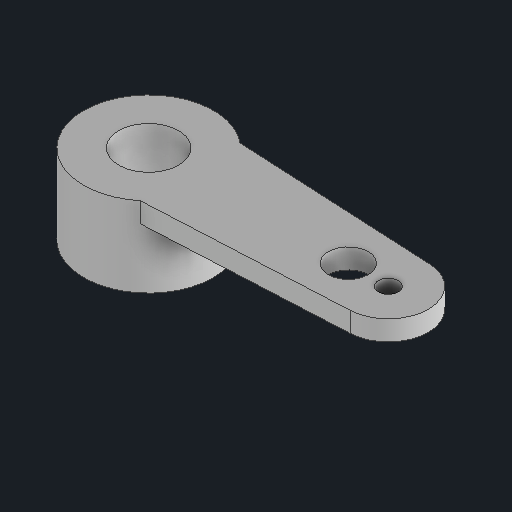
# Autodesk Inventor part: P_Servo_SIMPROP_lever
Saved by Autodesk Inventor 2026 (Build 300175000, 175)
## iProperties
Created: 2025-09-02
Part Number: P_Servo_SIMPROP_lever
Material: Generisch
Document SubType Name: Modeling
Designer: FAL
Density: 1 g/cm^3
Appearance: Vorgabe
Author: FAL
Autodesk Inventor part; units mm, degrees
ref_plane "YZ Plane" through (0, 0, 0) normal (1, 0, 0) x (0, 1, 0)
ref_plane "XZ Plane" through (0, 0, 0) normal (0, 1, 0) x (-1, 0, 0)
ref_plane "XY Plane" through (0, 0, 0) normal (0, 0, 1) x (1, 0, 0)
sketch "Skizze1" plane through (0, 0, 0) normal (0, 0, 1) x (1, 0, 0)
  circle A0 centre (0, 0) radius 3.25
  circle A1 centre (12, 0) radius 2
  line L0 (0, 0) -> (12, 0) construction
  line L1 (12.1001, 1.9975) -> (2.0767, 2.5)
  line L2 (2.0767, -2.5) -> (12.1001, -1.9975)
  dimension "d0" = 6.5
  dimension "d1" = 12
  dimension "d2" = 4
  dimension "d3" = 2.5
  dimension "d4" = 2.5
  constraints: 6 end point, 4 point on circle, 2 centre point, 2 tangent, 1 coincident, 1 horizontal
  measures "d0" diameter of A0
  measures "d1" distance of L0.start L0.end
  measures "d2" diameter of A1
  measures "d3" distance from line of L0 L1.end
  measures "d4" distance from line of L0 L2.start
extrude "Extrusion1" add sketch "Skizze1" along normal blind 1
sketch "Skizze2" plane through (0, 0, 0) normal (0, 0, -1) x (-1, 0, 0)
  line L0 (-2.0767, -2.5) -> (-12.1001, -1.9975) projected
  circle A0 centre (0, 0) radius 3.25
  constraints: 1 coincident, 3 other
extrude "Extrusion2" add sketch "Skizze2" along normal blind 3
sketch "Skizze3" plane through (0, 0, 1) normal (0, 0, 1) x (1, 0, 0)
  arc A0 (12.1001, -1.9975) -> (12.1001, 1.9975) centre (12, 0) ccw projected
  circle A1 centre (12, 0) radius 0.5
  circle A2 centre (10, 0) radius 1
  point P0 (0, 0)
  dimension "d9" = 2
  dimension "d10" = 1
  dimension "d11" = 2
  constraints: 2 centre point, 1 coincident, 1 horizontal alignment
  measures "d9" diameter of A2
  measures "d10" diameter of A1
  measures "d11" distance of A1.centre A2.centre
extrude "Extrusion3" cut sketch "Skizze3" against normal blind 3.25
sketch "Skizze4" plane through (0, 0, 1) normal (0, 0, 1) x (1, 0, 0)
  circle A0 centre (0, 0) radius 1.5
  dimension "d14" = 3
  constraints: 1 centre point, 1 coincident
  measures "d14" diameter of A0
extrude "Extrusion4" cut sketch "Skizze4" against normal blind 6.25
